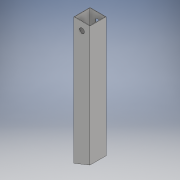
# Autodesk Inventor part: アッカーマンpipe1
Saved by Autodesk Inventor 2018 (Build 220112000, 112)
## iProperties
Created: 2017-09-17
Part Number: アッカーマンpipe1
Material: 一般
Document SubType Name: Modeling
Designer: Kenta
Density: 1 g/cm^3
Appearance: 既定
Author: Kenta
Autodesk Inventor part; units mm, degrees
ref_plane "YZ Plane" through (0, 0, 0) normal (1, 0, 0) x (0, 1, 0)
ref_plane "XZ Plane" through (0, 0, 0) normal (0, 1, 0) x (-1, 0, 0)
ref_plane "XY Plane" through (0, 0, 0) normal (0, 0, 1) x (1, 0, 0)
sketch "スケッチ1" plane through (0, 0, 0) normal (0, 0, 1) x (1, 0, 0)
  point P0 (0, 0)
sketch "スケッチ2" plane through (0, 0, 0) normal (0, 0, 1) x (1, 0, 0)
  line L0 (-16, 16) -> (16, 16)
  line L1 (16, 16) -> (16, -16)
  line L2 (16, -16) -> (-16, -16)
  line L3 (-16, -16) -> (-16, 16)
  line L4 (-16, 16) -> (16, -16) construction
  line L5 (16, 16) -> (-16, -16) construction
  line L6 (-15.2, 15.2) -> (15.2, 15.2)
  line L7 (15.2, 15.2) -> (15.2, -15.2)
  line L8 (15.2, -15.2) -> (-15.2, -15.2)
  line L9 (-15.2, -15.2) -> (-15.2, 15.2)
  line L10 (-15.2, 15.2) -> (15.2, -15.2) construction
  line L11 (15.2, 15.2) -> (-15.2, -15.2) construction
  point P0 (0, 0)
  point P1 (0, 0)
  dimension "d0" = 32
  dimension "d1" = 32
  dimension "d2" = 30.4
  dimension "d3" = 30.4
  constraints: 24 end point, 6 midpoint, 4 parallel, 2 horizontal, 2 perpendicular
  measures "d0" distance of L1.end L2.end
  measures "d1" distance of L0.end L1.end
  measures "d2" distance of L7.end L8.end
  measures "d3" distance of L6.end L7.end
extrude "押し出し1" add sketch "スケッチ2" along normal blind 251.7399
sketch "スケッチ3" plane through (-16, 16, 0) normal (0, 1, 0) x (1, 0, 0)
  line L0 (32, -251.7399) -> (0, -251.7399) projected
  point P0 (16, 0)
  point P1 (16, -235.7399)
  dimension "d6" = 16
  measures "d6" distance from line of L0 point (16, -235.74)
hole "穴1" at (0, 16, 235.7399) direction (0, -1, 0) diameter 10 end through all
sketch "スケッチ4" plane through (-16, 16, 0) normal (0, 1, 0) x (1, 0, 0)
  point P0 (16, 0)
sketch "スケッチ5" plane through (-16, 16, 0) normal (0, 1, 0) x (1, 0, 0)
  line L0 (0, 0) -> (32, -12.9008)
  line L1 (32, 0) -> (32, -251.7399) projected
  line L2 (0, 0) -> (34.5026, 0) construction
  line L3 (32, -12.9008) -> (32, 0)
  line L4 (0, 0) -> (32, 0) projected
  line L5 (32, 0) -> (0, 0)
  point P0 (16, 0)
  dimension "d14" = 21.957
  constraints: 8 end point, 1 collinear, 1 equal length, 1 horizontal, 1 perpendicular, 1 point on line
  measures "d14" angle of L0 L2
extrude "押し出し2" cut sketch "スケッチ5" against normal blind 32
